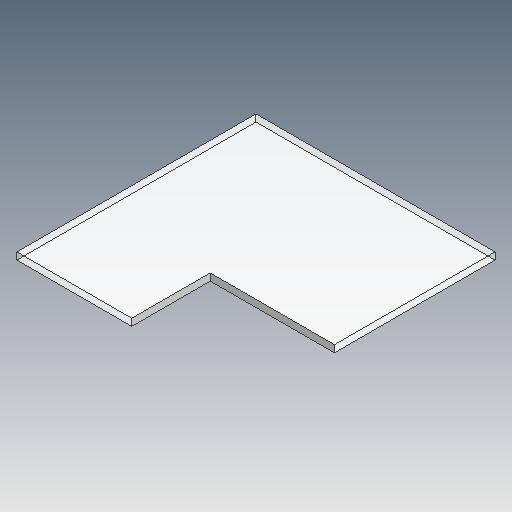
# Autodesk Inventor part: acrylic_cover
Saved by Autodesk Inventor 2025.4 (Build 294407020, 407B)
## iProperties
Created: 2026-09-08
Part Number: acrylic_cover
Material: Generic
Document SubType Name: Modeling
Designer: Aiden
Density: 1 g/cm^3
Appearance: Default
Author: Aiden
Autodesk Inventor part; units mm, degrees
ref_plane "YZ Plane" through (0, 0, 0) normal (1, 0, 0) x (0, 1, 0)
ref_plane "XZ Plane" through (0, 0, 0) normal (0, 1, 0) x (-1, 0, 0)
ref_plane "XY Plane" through (0, 0, 0) normal (0, 0, 1) x (1, 0, 0)
sketch "Sketch1" plane through (0, 0, 0) normal (0, 1, 0) x (-1, 0, 0)
  line L0 (0, 0) -> (-304.8, 0)
  line L1 (-304.8, 0) -> (-304.8, -304.8)
  line L2 (-304.8, -304.8) -> (0, -304.8)
  line L3 (0, -304.8) -> (0, 0)
  dimension "d0" = 304.8
  dimension "d1" = 304.8
  constraints: 8 end point, 2 parallel, 1 horizontal, 1 perpendicular
  measures "d0" distance of L1.end L2.end
  measures "d1" distance of L2.end L0.start
extrude "Extrusion1" add sketch "Sketch1" along normal blind 9
sketch "Sketch3" plane through (0, 9, 0) normal (0, 1, 0) x (1, 0, 0)
  line L0 (197.0873, 95) -> (302.0873, 95) projected
  line L1 (302.0873, 18.175) -> (197.0873, 18.175) projected
  line L2 (153.4243, 27.425) -> (153.4243, 72.575) projected
  line L3 (304.8, 0) -> (304.8, 304.8) projected
  line L4 (304.8, 100) -> (146.4243, 100)
  line L5 (146.4243, 100) -> (146.4243, 0)
  line L6 (146.4243, 0) -> (304.8, 0)
  line L7 (304.8, 0) -> (304.8, 100)
  point P0 (0, 0)
  dimension "d8" = 5
  dimension "d9" = 7
  constraints: 8 end point, 2 perpendicular, 1 collinear, 1 horizontal, 1 point on line
  measures "d8" distance between parallel lines of L4 L0
  measures "d9" distance between parallel lines of L5 L2
extrude "Extrusion3" cut sketch "Sketch3" against normal blind 10
sketch "Sketch2" plane through (0, 9, 0) normal (0, 1, 0) x (1, 0, 0)
  line L0 (304.8, 304.8) -> (0, 304.8) projected
  line L1 (304.8, 304.8) -> (144.8, 304.8)
  line L2 (144.8, 304.8) -> (144.8, 209.8)
  line L3 (144.8, 209.8) -> (304.8, 209.8)
  line L4 (304.8, 209.8) -> (304.8, 304.8)
  point P0 (0, 0)
  dimension "d4" = 95
  dimension "d5" = 160
  constraints: 8 end point, 2 parallel, 1 horizontal, 1 perpendicular
  measures "d4" distance of L1.end L2.end
  measures "d5" distance of L2.end L3.end
body "Solid1"
